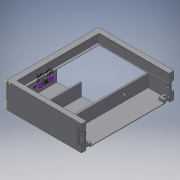
# Autodesk Inventor part: Bauteil1
Saved by Autodesk Inventor 2016 SP2 (Build 200236200, 236)
## iProperties
Created: 2018-06-21
Part Number: Bauteil1
Material: Generisch
Document SubType Name: Modeling
Designer: Nils
Density: 1 g/cm^3
Appearance: Vorgabe
Author: Nils
Autodesk Inventor part; units mm, degrees
ref_plane "YZ Plane" through (0, 0, 0) normal (1, 0, 0) x (0, 1, 0)
ref_plane "XZ Plane" through (0, 0, 0) normal (0, 1, 0) x (-1, 0, 0)
ref_plane "XY Plane" through (0, 0, 0) normal (0, 0, 1) x (1, 0, 0)
sketch "Skizze1" plane through (0, 0, 0) normal (0, 0, 1) x (1, 0, 0)
  line L0 (0, 0) -> (137.4, 0)
  line L1 (137.4, 0) -> (137.4, 9)
  line L2 (137.4, 9) -> (10, 9)
  line L3 (10, 9) -> (10, 159.5)
  line L4 (10, 159.5) -> (137.4, 159.5)
  line L5 (137.4, 159.5) -> (137.4, 168.5)
  line L6 (137.4, 168.5) -> (0, 168.5)
  line L7 (0, 168.5) -> (0, 0)
  dimension "d0" = 9
  dimension "d1" = 9
  dimension "d2" = 150.5
  dimension "d3" = 10
  dimension "d4" = 137.4
  constraints: 16 end point, 6 perpendicular, 2 point on line, 1 horizontal
  measures "d0" distance of L0.end L1.end
  measures "d1" distance of L4.end L5.end
  measures "d2" distance of L2.end L3.end
  measures "d3" distance between parallel lines of L7 L3
  measures "d4" distance of L0.start L0.end
extrude "Extrusion1" add sketch "Skizze1" along normal blind 1
sketch "Skizze2" plane through (0, 0, 0) normal (0, 0, -1) x (-1, 0, 0)
  line L0 (0, 0) -> (-137.4, 0) projected
  line L1 (0, 168.5) -> (0, 0) projected
  line L2 (-137.4, 168.5) -> (0, 168.5) projected
  line L3 (-137.4, 0) -> (-137.4, 4.5)
  line L4 (-137.4, 0) -> (-137.4, 9) projected
  line L5 (-6, 7.5) -> (-6, 161)
  line L6 (-10, 9) -> (-10, 159.5) projected
  line L7 (-6, 161) -> (-137.4, 161)
  line L8 (-137.4, 159.5) -> (-137.4, 168.5) projected
  line L9 (-137.4, 161) -> (-137.4, 168.5)
  line L10 (-10, 159.5) -> (-137.4, 159.5) projected
  line L11 (-6, 7.5) -> (-137.4, 7.5)
  line L12 (0, 0) -> (-137.4, 0) projected
  line L13 (-137.4, 7.5) -> (-137.4, 0)
  line L14 (-137.4, 9) -> (-10, 9) projected
  dimension "d7" = 1.5
  dimension "d8" = 1.5
  dimension "d9" = 4
  constraints: 12 end point, 2 parallel, 2 perpendicular, 2 point on line, 1 collinear, 1 midpoint
  measures "d7" distance between parallel lines of L10 L7
  measures "d8" distance between parallel lines of L14 L11
  measures "d9" distance between parallel lines of L6 L5
extrude "Extrusion2" add sketch "Skizze2" along normal blind 17 contours L0 L3 L4 L11 L5 L7 L8 L2 L1
sketch "Skizze3" plane through (0, 0, -17) normal (0, 0, -1) x (-1, 0, 0)
  line L0 (0, 0) -> (-137.4, 0) projected
  line L1 (-137.4, 0) -> (-137.4, 9) projected
  line L2 (-137.4, 9) -> (-10, 9) projected
  line L3 (-10, 9) -> (-10, 159.5) projected
  line L4 (-10, 159.5) -> (-137.4, 159.5) projected
  line L5 (-137.4, 159.5) -> (-137.4, 168.5) projected
  line L6 (-137.4, 168.5) -> (0, 168.5) projected
  line L7 (0, 168.5) -> (0, 0) projected
extrude "Extrusion3" add sketch "Skizze3" along normal blind 2
sketch "Skizze4" plane through (0, 0, -19) normal (0, 0, -1) x (-1, 0, 0)
  line L0 (-6, 161) -> (-137.4, 161) projected
  line L1 (-137.4, 161) -> (-6, 161) projected
  line L2 (-6, 7.5) -> (-6, 161) projected
  line L3 (-6, 161) -> (-6, 7.5) projected
  line L4 (-137.4, 7.5) -> (-6, 7.5) projected
  line L5 (-6, 7.5) -> (-137.4, 7.5) projected
  line L6 (0, 168.5) -> (-137.4, 168.5) projected
  line L7 (0, 0) -> (0, 168.5) projected
  line L8 (-137.4, 0) -> (0, 0) projected
  line L9 (0, 0) -> (-137.4, 0) projected
  line L10 (-137.4, 0) -> (-137.4, 7.5)
  line L11 (-137.4, 168.5) -> (-137.4, 159.5) projected
  line L12 (-137.4, 161) -> (-137.4, 168.5)
  line L13 (-137.4, 161) -> (-6, 161)
  line L14 (-6, 161) -> (-6, 7.5) projected
  line L15 (-6, 161) -> (-6, 7.5)
  line L16 (-137.4, 7.5) -> (-6, 7.5) projected
  line L17 (-6, 7.5) -> (-137.4, 7.5)
  constraints: 10 end point, 3 collinear, 2 perpendicular
extrude "Extrusion4" add sketch "Skizze4" along normal blind 23
sketch "Skizze5" plane through (0, 0, -42) normal (0, 0, -1) x (-1, 0, 0)
  line L0 (-137.4, 159.5) -> (-137.4, 168.5) projected
  line L1 (0, 0) -> (-137.4, 0) projected
  line L2 (-137.4, 168.5) -> (0, 168.5)
  line L3 (0, 168.5) -> (0, 0)
  line L4 (0, 0) -> (-137.4, 0)
  line L5 (-137.4, 0) -> (-137.4, 168.5)
  constraints: 8 end point, 2 parallel, 1 horizontal, 1 perpendicular
extrude "Extrusion5" add sketch "Skizze5" along normal blind 3
sketch "Skizze6" plane through (6, 7.5, -19) normal (0, 1, 0) x (1, 0, 0)
  line L0 (0, 0) -> (0, 23) projected
  line L1 (131.4, 0) -> (0, 0) projected
  line L2 (43.5, 0) -> (45.5, 0)
  line L3 (45.5, 0) -> (45.5, 23)
  line L4 (45.5, 23) -> (43.5, 23)
  line L5 (43.5, 23) -> (43.5, 0)
  line L6 (0, 23) -> (131.4, 23) projected
  line L7 (89, 23) -> (92, 23)
  line L8 (92, 23) -> (92, 0)
  line L9 (92, 0) -> (89, 0)
  line L10 (89, 0) -> (89, 23)
  point P0 (-6, -19)
  dimension "d24" = 43.5
  dimension "d25" = 43.5
  dimension "d26" = 2
  dimension "d27" = 3
  constraints: 16 end point, 4 parallel, 3 point on line, 2 horizontal, 2 perpendicular
  measures "d24" distance between parallel lines of L5 L0
  measures "d25" distance between parallel lines of L10 L3
  measures "d26" distance between parallel lines of L3 L5
  measures "d27" distance between parallel lines of L8 L10
chamfer "Fase2" distance 1.5 angle 45 2 edges at (73.7, 159.5, -19) (73.7, 9, -19)
chamfer "Fase3" distance 1.5 angle 45 1 edges at (10, 84.25, -19)
extrude "Extrusion7" add sketch "Skizze6" along normal blind 78.5 contours L5 L4 L3 L1 | L10 L6 L8 L1
sketch "Skizze7" plane through (0, 0, -42) normal (0, 0, 1) x (1, 0, 0)
  line L0 (137.4, 159.5) -> (10, 159.5) projected
  line L1 (98, 86) -> (96, 86)
  line L2 (137.4, 161) -> (6, 161) projected
  line L3 (98, 86) -> (95.5, 86)
  line L4 (95.5, 86) -> (95.5, 161)
  line L5 (95.5, 161) -> (98, 161)
  line L6 (98, 161) -> (98, 86)
  point P0 (0, 0)
  dimension "d46" = 2.5
  constraints: 10 end point, 2 horizontal, 2 parallel, 1 coincident, 1 perpendicular, 1 point on line
  measures "d46" distance of L4.end L5.end
extrude "Extrusion8" add sketch "Skizze7" along normal blind 23
sketch "Skizze8" plane through (0, 168.5, 1) normal (0, 1, 0) x (1, 0, 0)
  line L0 (95.5, 20) -> (95.5, 41) projected
  line L1 (0, 46) -> (95.5, 46)
  line L2 (95.5, 46) -> (95.5, 20)
  line L3 (95.5, 20) -> (0, 20)
  line L4 (0, 20) -> (0, 46)
  point P0 (0, 1)
  constraints: 8 end point, 2 parallel, 1 horizontal, 1 perpendicular
extrude "Extrusion9" cut sketch "Skizze8" against normal blind 82.5
sketch "Skizze9" plane through (95.5, 86, -45) normal (-1, 0, 0) x (0, 0, 1)
  line L0 (3, 0) -> (26, 0) projected
  line L1 (3, 0) -> (3, 1)
  line L2 (3, 75) -> (3, -78.5) projected
  line L3 (3, 1) -> (1, 1)
  line L4 (1, 1) -> (2, 0)
  line L5 (26, 0) -> (0, 0) projected
  line L6 (2, 0) -> (3, 0)
  point P0 (45, -86)
  dimension "d47" = 2
  dimension "d48" = 1
  dimension "d49" = 1
  constraints: 8 end point, 2 point on line, 1 collinear, 1 horizontal
  measures "d47" distance of L1.end L3.end
  measures "d48" distance of L0.start L1.end
  measures "d49" distance from line of L4.end L1
extrude "Extrusion10" add sketch "Skizze9" along normal blind 89.5
sketch "Skizze10" plane through (95.5, 86, -45) normal (-1, 0, 0) x (0, 0, 1)
  line L0 (26, 82.5) -> (26, 75) projected
  line L1 (26, 80.5) -> (25, 81.5)
  line L2 (25, 81.5) -> (25, 79.5)
  line L3 (25, 79.5) -> (26, 78.5)
  line L4 (26, 78.5) -> (26, 80.5)
  line L5 (0, 82.5) -> (26, 82.5) projected
  point P0 (45, -86)
  dimension "d52" = 2
  dimension "d53" = 1
  dimension "d54" = 2
  dimension "d55" = 1
  constraints: 8 end point, 2 parallel, 1 collinear, 1 point on line
  measures "d52" distance of L1.end L2.end
  measures "d53" distance from line of L0 L1.end
  measures "d54" distance of L1.start L0.start
  measures "d55" distance from line of L5 L1.end
extrude "Extrusion11" add sketch "Skizze10" along normal blind 89.5
sketch "Skizze11" plane through (0, 0, 1) normal (0, -1, 0) x (1, 0, 0)
  line L0 (0, 0) -> (137.4, 0) construction
  line L1 (129.4, 0) -> (129.4, -46) construction
  line L2 (95.5, -46) -> (137.4, -46) construction
  line L3 (137.4, -46) -> (137.4, 0) projected
  line L4 (137.4, -15) -> (129.4, -7)
  line L5 (129.4, -7) -> (129.4, -39)
  line L6 (129.4, -39) -> (137.4, -31)
  point P0 (0, -1)
  dimension "d58" = 15
  dimension "d59" = 15
  dimension "d60" = 8
  dimension "d61" = 8
  dimension "d62" = 8
  dimension "d63" = 16
  constraints: 8 end point, 6 point on line, 1 vertical
  measures "d58" distance of L2.end L6.end
  measures "d59" distance of L0.end L4.start
  measures "d60" distance between parallel lines of L1 L3
  measures "d61" horizontal distance of L5.end L6.end
  measures "d62" horizontal distance of L4.end L4.start
  measures "d63" distance of L6.end L4.start
extrude "Extrusion12" cut sketch "Skizze11" against normal blind 4.5
sketch "Skizze13" plane through (0, 4.5, 1) normal (0, -1, 0) x (1, 0, 0)
  line L0 (137.4, -15) -> (137.4, -31) projected
  line L1 (129.4, -7) -> (137.4, -15) projected
  line L2 (129.4, -39) -> (129.4, -7) projected
  line L3 (137.4, -31) -> (129.4, -39) projected
  line L4 (137.4, -20) -> (137.4, -43) construction
  line L5 (137.4, -23) -> (129.4, -23) construction
  circle A0 centre (133.4, -23) radius 1.75
  point P0 (0, -1)
  dimension "d66" = 3.5
  constraints: 2 end point, 2 midpoint, 1 centre point, 1 perpendicular, 1 point on line
  measures "d66" diameter of A0
extrude "Extrusion13" cut sketch "Skizze13" against normal blind 4.5 contours A0
sketch "Skizze14" plane through (137.4, 7.5, -19) normal (0, 1, 0) x (1, 0, 0)
  circle A0 centre (-4, 3) radius 1.75 construction
  line L0 (-5.6166, 5.8) -> (-2.3834, 5.8)
  line L1 (-2.3834, 5.8) -> (-0.7668, 3)
  line L2 (-0.7668, 3) -> (-2.3834, 0.2)
  line L3 (-2.3834, 0.2) -> (-5.6166, 0.2)
  line L4 (-5.6166, 0.2) -> (-7.2332, 3)
  line L5 (-7.2332, 3) -> (-5.6166, 5.8)
  point P0 (-137.4, -19)
  dimension "d69" = 5.6
  constraints: 12 end point, 1 coincident, 1 horizontal, 13 other
  measures "d69" distance between parallel lines of L2 L5
extrude "Extrusion14" cut sketch "Skizze14" against normal blind 2
chamfer "Fase4" distance 2 angle 5 1 edges at (130.9751, 7.5, -20.6) measured on face at (131.2446, 6.8333, -20.1333)
chamfer "Fase5" distance 2 angle 5 1 edges at (130.9751, 7.5, -23.4) measured on face at (131.2446, 6.1668, -23.8667)
chamfer "Fase6" distance 2 angle 5 1 edges at (133.4, 7.5, -24.8) measured on face at (133.9389, 6.1668, -24.8)
chamfer "Fase7" distance 2 angle 5 1 edges at (135.8249, 7.5, -23.4) measured on face at (136.0943, 6.1668, -22.9333)
chamfer "Fase9" distance 2 angle 5 1 edges at (133.4, 7.5, -19.2) measured on face at (133.9389, 6.1668, -19.2)
chamfer "Fase20" distance 2 angle 5 1 edges at (135.8249, 7.5, -20.6) measured on face at (136.0943, 6.167, -21.0667)
sketch "Skizze15" plane through (98, 7.5, -19) normal (1, 0, 0) x (0, 0, -1)
  line L0 (9, 108.5) -> (14, 108.5)
  line L1 (14, 108.5) -> (14, 113.5)
  line L2 (14, 113.5) -> (9, 113.5)
  line L3 (9, 113.5) -> (9, 108.5)
  line L4 (0, 153.5) -> (23, 153.5) projected
  line L5 (0, 153.5) -> (0, 78.5) projected
  point P0 (-19, -7.5)
  dimension "d90" = 5
  dimension "d91" = 5
  dimension "d92" = 40
  dimension "d93" = 9
  constraints: 8 end point, 2 parallel, 1 horizontal, 1 perpendicular
  measures "d90" distance of L2.end L1.end
  measures "d91" distance of L1.end L0.end
  measures "d92" distance from line of L4 L1.end
  measures "d93" distance between parallel lines of L5 L3
extrude "Extrusion15" cut sketch "Skizze15" against normal blind 40
sketch "Skizze16" plane through (0, 168.5, 1) normal (0, 1, 0) x (1, 0, 0)
  circle A0 centre (133.4, 23) radius 1.75 projected
  line L0 (137.4, 15) -> (137.4, 31) projected
  line L1 (129.4, 7) -> (137.4, 15) projected
  line L2 (129.4, 39) -> (129.4, 7) projected
  line L3 (137.4, 31) -> (129.4, 39) projected
  point P0 (0, 1)
extrude "Extrusion16" cut sketch "Skizze16" against normal blind 4.5
sketch "Skizze17" plane through (133.4, 168.5, -22) normal (0, 1, 0) x (1, 0, 0)
  circle A0 centre (0, 0) radius 1.75 projected
  point P0 (-133.4, -22)
extrude "Extrusion17" cut sketch "Skizze17" against normal blind 18
sketch "Skizze19" plane through (137.4, 161, -42) normal (0, -1, 0) x (1, 0, 0)
  circle A0 centre (-4, 20) radius 1.75 projected
  line L0 (-5.6166, 17.2) -> (-2.3834, 17.2) projected
  line L1 (-7.2332, 20) -> (-5.6166, 17.2) projected
  line L2 (-5.6166, 22.8) -> (-7.2332, 20) projected
  line L3 (-2.3834, 22.8) -> (-5.6166, 22.8) projected
  line L4 (-0.7668, 20) -> (-2.3834, 22.8) projected
  line L5 (-2.3834, 17.2) -> (-0.7668, 20) projected
  point P0 (-137.4, 42)
extrude "Extrusion18" cut sketch "Skizze19" against normal blind 2
chamfer "Fase14" distance 2 angle 5 1 edges at (130.9751, 161, -20.6) measured on face at (130.7057, 162.3333, -21.0667)
chamfer "Fase15" distance 2 angle 5 1 edges at (133.4, 161, -19.2) measured on face at (133.9389, 162.3332, -19.2)
chamfer "Fase16" distance 2 angle 5 1 edges at (135.8249, 161, -20.6) measured on face at (136.0943, 162.3332, -21.0667)
chamfer "Fase17" distance 2 angle 5 1 edges at (135.8249, 161, -23.4) measured on face at (135.5554, 162.3332, -23.8667)
chamfer "Fase18" distance 2 angle 5 1 edges at (133.4, 161, -24.8) measured on face at (132.8611, 162.3332, -24.8)
chamfer "Fase19" distance 2 angle 5 1 edges at (130.9751, 161, -23.4) measured on face at (130.7057, 161.6665, -22.9333)
sketch "Skizze21" plane through (0, 0, -45) normal (0, 0, -1) x (-1, 0, 0)
  line L0 (-98, 7.5) -> (-137.4, 7.5) projected
  line L1 (-137.4, 7.5) -> (-129.4, 7.5)
  line L2 (-129.4, 7.5) -> (-129.4, 161)
  line L3 (-6, 161) -> (-137.4, 161) projected
  line L4 (-137.4, 161) -> (-129.4, 161)
  line L5 (-137.4, 161) -> (-137.4, 7.5)
  point P0 (0, 0)
  dimension "d137" = 8
  constraints: 8 end point, 2 point on line, 1 collinear, 1 parallel, 1 perpendicular
  measures "d137" distance of L0.end L1.end
extrude "Extrusion20" cut sketch "Skizze21" against normal blind 2
sketch "Skizze22" plane through (0, 0, -42) normal (0, 0, 1) x (1, 0, 0)
  line L0 (137.4, 7.5) -> (127.4, 7.5)
  line L1 (127.4, 7.5) -> (127.4, 17.5)
  line L2 (127.4, 17.5) -> (137.4, 17.5)
  line L3 (137.4, 17.5) -> (137.4, 7.5)
  line L4 (137.4, 161) -> (127.4, 161)
  line L5 (127.4, 161) -> (127.4, 151)
  line L6 (127.4, 151) -> (137.4, 151)
  line L7 (137.4, 151) -> (137.4, 161)
  point P0 (0, 0)
  dimension "d140" = 10
  dimension "d141" = 10
  dimension "d142" = 10
  dimension "d143" = 10
  constraints: 16 end point, 4 parallel, 2 horizontal, 2 perpendicular
  measures "d140" distance of L1.end L2.end
  measures "d141" distance of L0.end L1.end
  measures "d142" distance of L6.end L5.end
  measures "d143" distance of L5.end L4.end
extrude "Extrusion21" add sketch "Skizze22" along normal blind 5
sketch "Skizze23" plane through (0, 0, -43) normal (0, 0, -1) x (-1, 0, 0)
  line L0 (-129.4, 161) -> (-129.4, 7.5) projected
  line L1 (-129.4, 7.5) -> (-137.4, 7.5)
  line L2 (-137.4, 7.5) -> (-137.4, 15.5)
  line L3 (-137.4, 15.5) -> (-129.4, 15.5)
  line L4 (-129.4, 15.5) -> (-129.4, 7.5)
  line L5 (-129.4, 161) -> (-137.4, 161)
  line L6 (-137.4, 161) -> (-137.4, 153)
  line L7 (-137.4, 153) -> (-129.4, 153)
  line L8 (-129.4, 153) -> (-129.4, 161)
  point P0 (0, 0)
  dimension "d146" = 8
  dimension "d147" = 8
  dimension "d148" = 8
  dimension "d149" = 8
  constraints: 16 end point, 4 parallel, 2 horizontal, 2 perpendicular
  measures "d146" distance of L2.end L3.end
  measures "d147" distance of L1.end L2.end
  measures "d148" distance of L7.end L6.end
  measures "d149" distance of L6.end L5.end
extrude "Extrusion22" cut sketch "Skizze23" against normal blind 2.5
sketch "Skizze24" plane through (0, 0, -40.5) normal (0, 0, -1) x (-1, 0, 0)
  line L0 (-137.4, 161) -> (-129.4, 161) projected
  line L1 (-137.4, 153) -> (-137.4, 161) projected
  line L2 (-129.4, 153) -> (-137.4, 153) projected
  line L3 (-129.4, 161) -> (-129.4, 153) projected
  line L4 (-129.4, 15.5) -> (-129.4, 7.5) projected
  line L5 (-137.4, 15.5) -> (-129.4, 15.5) projected
  line L6 (-137.4, 7.5) -> (-137.4, 15.5) projected
  line L7 (-129.4, 7.5) -> (-137.4, 7.5) projected
  line L8 (-137.4, 7.5) -> (-129.4, 15.5) construction
  line L9 (-137.4, 161) -> (-129.4, 153) construction
  circle A0 centre (-133.4, 157) radius 1.75
  circle A1 centre (-133.4, 11.5) radius 1.75
  point P0 (0, 0)
  dimension "d152" = 3.5
  dimension "d153" = 3.5
  constraints: 4 end point, 2 centre point, 2 midpoint, 1 perpendicular
  measures "d152" diameter of A0
  measures "d153" diameter of A1
extrude "Extrusion23" cut sketch "Skizze24" against normal blind 4.5 contours A0 | A1
sketch "Skizze25" plane through (0, 0, -37) normal (0, 0, 1) x (1, 0, 0)
  circle A0 centre (133.4, 157) radius 1.75 projected
  line L0 (136.3, 158.6743) -> (136.3, 155.3257)
  line L1 (136.3, 155.3257) -> (133.4, 153.6514)
  line L2 (133.4, 153.6514) -> (130.5, 155.3257)
  line L3 (130.5, 155.3257) -> (130.5, 158.6743)
  line L4 (130.5, 158.6743) -> (133.4, 160.3486)
  line L5 (133.4, 160.3486) -> (136.3, 158.6743)
  circle A1 centre (133.4, 11.5) radius 1.75 projected
  line L6 (130.5, 13.1743) -> (133.4, 14.8486)
  line L7 (133.4, 14.8486) -> (136.3, 13.1743)
  line L8 (136.3, 13.1743) -> (136.3, 9.8257)
  line L9 (136.3, 9.8257) -> (133.4, 8.1514)
  line L10 (133.4, 8.1514) -> (130.5, 9.8257)
  line L11 (130.5, 9.8257) -> (130.5, 13.1743)
  point P0 (0, 0)
  dimension "d156" = 5.8
  dimension "d157" = 5.8
  constraints: 24 end point, 2 coincident, 2 vertical, 26 other
  measures "d156" distance between parallel lines of L0 L3
  measures "d157" distance between parallel lines of L8 L11
extrude "Extrusion24" cut sketch "Skizze25" against normal blind 2.5
sketch "Skizze26" plane through (0, 0, 1) normal (-1, 0, 0) x (0, 0, 1)
  line L0 (-43, 86) -> (-20, 86) projected
  line L1 (-20, 86) -> (-46, 86) construction
  line L2 (-33, 86) -> (-33, 0) construction
  line L3 (-46, 0) -> (-31, 0) construction
  circle A0 centre (-33, 76) radius 1.75
  circle A1 centre (-33, 56) radius 1.75
  point P0 (-1, 0)
  dimension "d160" = 3.5
  dimension "d161" = 3.5
  dimension "d162" = 10
  dimension "d163" = 20
  constraints: 3 point on line, 2 centre point, 2 end point, 1 midpoint, 1 vertical
  measures "d160" diameter of A0
  measures "d161" diameter of A1
  measures "d162" distance from line of L0 A0.centre
  measures "d163" distance of A1.centre A0.centre
sketch "Skizze27" plane through (6, 7.5, -19) normal (1, 0, 0) x (0, 0, -1)
  circle A0 centre (13, 68.5) radius 1.75 projected
  circle A1 centre (13, 48.5) radius 1.75 projected
  line L0 (10.1, 66.8257) -> (10.1, 70.1743)
  line L1 (10.1, 70.1743) -> (13, 71.8486)
  line L2 (13, 71.8486) -> (15.9, 70.1743)
  line L3 (15.9, 70.1743) -> (15.9, 66.8257)
  line L4 (15.9, 66.8257) -> (13, 65.1514)
  line L5 (13, 65.1514) -> (10.1, 66.8257)
  line L6 (10.1, 46.8257) -> (10.1, 50.1743)
  line L7 (10.1, 50.1743) -> (13, 51.8486)
  line L8 (13, 51.8486) -> (15.9, 50.1743)
  line L9 (15.9, 50.1743) -> (15.9, 46.8257)
  line L10 (15.9, 46.8257) -> (13, 45.1514)
  line L11 (13, 45.1514) -> (10.1, 46.8257)
  point P0 (-19, -7.5)
  dimension "d166" = 5.8
  dimension "d167" = 5.8
  constraints: 24 end point, 2 coincident, 2 vertical, 26 other
  measures "d166" distance between parallel lines of L9 L6
  measures "d167" distance between parallel lines of L3 L0
sketch "Skizze28" plane through (0, 0, 1) normal (-1, 0, 0) x (0, 0, 1)
  line L0 (0, 0) -> (-46, 0) construction
  line L1 (-23, 0) -> (-23, 86) construction
  line L2 (-43, 86) -> (-20, 86) construction
  circle A0 centre (-23, 76) radius 5
  circle A1 centre (-23, 51) radius 5
  point P0 (-1, 0)
  dimension "d170" = 10
  dimension "d171" = 10
  dimension "d172" = 10
  dimension "d173" = 25
  constraints: 3 point on line, 2 centre point, 2 end point, 1 midpoint, 1 vertical
  measures "d170" diameter of A0
  measures "d171" diameter of A1
  measures "d172" distance from line of L2 A0.centre
  measures "d173" distance of A1.centre A0.centre
extrude "Extrusion27" cut sketch "Skizze28" against normal blind 5
thread "Gewinde3" size "M10x1.5" class "6H" standard "ANSI Metric M Profile" full length
thread "Gewinde4" size "M10x1.5" class "6H" standard "ANSI Metric M Profile" full length
sketch "Skizze34" plane through (5, 51, -22) normal (0, -1, 0) x (0, 0, 1)
  line L0 (5, 0) -> (5, 5)
  line L1 (5, 5) -> (4.0211, 5)
  line L2 (4.0211, 5) -> (4.0211, 0)
  line L3 (4.0211, 0) -> (5, 0)
  line L4 (0, -159.88) -> (0, 32.48) projected
  constraints: 8 end point
revolve "Umdrehung3" add sketch "Skizze34" angle 360 about axis through (5, 51, -22) along (-1, 0, 0) separate body
sketch "Skizze33" plane through (5, 51, -17) normal (0, 1, 0) x (-1, 0, 0)
  line L0 (-0.8887, -0.0802) -> (-0.7501, -0.0802) construction
  line L1 (0.1385, -0.899) -> (-0.0001, -1.1391) construction
  line L2 (-1.5001, -1.1391) -> (-1.6387, -0.899) construction
  line L3 (-0.6115, -0.0802) -> (-0.7501, 0.1599) construction
  line L4 (-0.7501, 0.1599) -> (-0.8887, -0.0802) construction
  line L5 (-1.5001, -1.1391) -> (-1.3615, -0.899) construction
  line L6 (-0.6115, -0.0802) -> (-0.1387, -0.899)
  line L7 (-1.6387, -0.899) -> (-1.3615, -0.899) construction
  arc A0 (-1.6387, -0.899) -> (-1.5001, -0.979) centre (-1.5001, -0.819) ccw construction
  line L8 (0.1385, -0.899) -> (-0.1387, -0.899) construction
  line L9 (-1.5001, -1.1391) -> (-1.5001, -0.899) construction
  line L10 (-0.0001, -1.1391) -> (-0.0001, -0.899) construction
  line L11 (-0.7501, 0.1599) -> (-0.7501, -0.0002) construction
  line L12 (-1.5001, -0.979) -> (-0.0001, -0.979)
  arc A1 (-1.5001, -0.979) -> (-1.3615, -0.899) centre (-1.5001, -0.819) ccw
  line L13 (-0.1387, -0.899) -> (-0.0001, -1.1391) construction
  line L14 (-1.3615, -0.899) -> (-0.8887, -0.0802)
  line L15 (-0.0001, -0.0002) -> (-0.0001, 0.0177)
  line L16 (-0.0001, 0.0177) -> (-0.0001, -0.0002)
  line L17 (-0.0001, -0.0002) -> (0.0334, -0.0002)
  arc A2 (-0.1387, -0.899) -> (-0.0001, -0.979) centre (-0.0001, -0.819) ccw
  arc A3 (-0.0001, -0.979) -> (0.1385, -0.899) centre (-0.0001, -0.819) ccw construction
  arc A4 (-0.7501, -0.0002) -> (-0.8887, -0.0802) centre (-0.7501, -0.1603) ccw
  arc A5 (-0.6115, -0.0802) -> (-0.7501, -0.0002) centre (-0.7501, -0.1603) ccw
  line L18 (-0.7501, -0.0002) -> (-0.7501, -0.0802) construction
  line L19 (-0.7501, -0.0802) -> (-0.6115, -0.0802) construction
  dimension "d220" = 60
  dimension "d221" = 0.2401
  dimension "d222" = 0.2401
  dimension "Skizze33_ThreadOffset" = 0
  dimension "Skizze33_MajorRadius" = 0.9789
  dimension "d225" = 1.5
  dimension "Skizze33_MinorRadius" = 0
  constraints: 40 end point, 12 point on circle, 10 parallel, 8 tangent, 6 centre point, 6 collinear, 2 midpoint, 2 point on line, 1 horizontal, 1 perpendicular, 3 other
  measures "d220" angle of L6 L14
  measures "d221" distance of L3.end L0.end
  measures "d222" distance of L1.end L10.end
  measures "Skizze33_ThreadOffset" distance between parallel lines of L15 L10
  measures "Skizze33_MajorRadius" distance from line of L12 L15.start
  measures "d225" distance from line of L1.end L9
  measures "Skizze33_MinorRadius" distance edge to line of A5 L17
coil "Spirale3" sketch "Skizze33" operation cut axis through (5, 51, -22) along (-1, 0, 0) pitch 1.5015 turns 5.328005 hand right bodies 2
sketch "Skizze36" plane through (5, 76, -22) normal (0, -1, 0) x (0, 0, 1)
  line L0 (5, 0) -> (5, 5)
  line L1 (5, 5) -> (4.0211, 5)
  line L2 (4.0211, 5) -> (4.0211, 0)
  line L3 (4.0211, 0) -> (5, 0)
  line L4 (0, -159.9745) -> (0, 33.0473) projected
  constraints: 8 end point
revolve "Umdrehung4" add sketch "Skizze36" angle 360 about axis through (5, 76, -22) along (-1, 0, 0) separate body
sketch "Skizze35" plane through (5, 76, -17) normal (0, 1, 0) x (-1, 0, 0)
  line L0 (-0.8887, -0.0802) -> (-0.7501, -0.0802) construction
  line L1 (0.1385, -0.899) -> (-0.0001, -1.1391) construction
  line L2 (-1.5001, -1.1391) -> (-1.6387, -0.899) construction
  line L3 (-0.6115, -0.0802) -> (-0.7501, 0.1599) construction
  line L4 (-0.7501, 0.1599) -> (-0.8887, -0.0802) construction
  line L5 (-1.5001, -1.1391) -> (-1.3615, -0.899) construction
  line L6 (-0.6115, -0.0802) -> (-0.1387, -0.899)
  line L7 (-1.6387, -0.899) -> (-1.3615, -0.899) construction
  arc A0 (-1.6387, -0.899) -> (-1.5001, -0.979) centre (-1.5001, -0.819) ccw construction
  line L8 (0.1385, -0.899) -> (-0.1387, -0.899) construction
  line L9 (-1.5001, -1.1391) -> (-1.5001, -0.899) construction
  line L10 (-0.0001, -1.1391) -> (-0.0001, -0.899) construction
  line L11 (-0.7501, 0.1599) -> (-0.7501, -0.0002) construction
  line L12 (-1.5001, -0.979) -> (-0.0001, -0.979)
  arc A1 (-1.5001, -0.979) -> (-1.3615, -0.899) centre (-1.5001, -0.819) ccw
  line L13 (-0.1387, -0.899) -> (-0.0001, -1.1391) construction
  line L14 (-1.3615, -0.899) -> (-0.8887, -0.0802)
  line L15 (-0.0001, -0.0002) -> (-0.0001, 0.0177)
  line L16 (-0.0001, 0.0177) -> (-0.0001, -0.0002)
  line L17 (-0.0001, -0.0002) -> (0.0334, -0.0002)
  arc A2 (-0.1387, -0.899) -> (-0.0001, -0.979) centre (-0.0001, -0.819) ccw
  arc A3 (-0.0001, -0.979) -> (0.1385, -0.899) centre (-0.0001, -0.819) ccw construction
  arc A4 (-0.7501, -0.0002) -> (-0.8887, -0.0802) centre (-0.7501, -0.1603) ccw
  arc A5 (-0.6115, -0.0802) -> (-0.7501, -0.0002) centre (-0.7501, -0.1603) ccw
  line L18 (-0.7501, -0.0002) -> (-0.7501, -0.0802) construction
  line L19 (-0.7501, -0.0802) -> (-0.6115, -0.0802) construction
  dimension "d238" = 60
  dimension "d239" = 0.2401
  dimension "d240" = 0.2401
  dimension "Skizze35_ThreadOffset" = 0
  dimension "Skizze35_MajorRadius" = 0.9789
  dimension "d243" = 1.5
  dimension "Skizze35_MinorRadius" = 0
  constraints: 40 end point, 12 point on circle, 10 parallel, 8 tangent, 6 centre point, 6 collinear, 2 midpoint, 2 point on line, 1 horizontal, 1 perpendicular, 3 other
  measures "d238" angle of L6 L14
  measures "d239" distance of L3.end L0.end
  measures "d240" distance of L1.end L10.end
  measures "Skizze35_ThreadOffset" distance between parallel lines of L15 L10
  measures "Skizze35_MajorRadius" distance from line of L12 L15.start
  measures "d243" distance from line of L1.end L9
  measures "Skizze35_MinorRadius" distance edge to line of A5 L17
coil "Spirale4" sketch "Skizze35" operation cut axis through (5, 76, -22) along (-1, 0, 0) pitch 1.5015 turns 5.328005 hand right bodies 3
equation "\"d1\" = d0"
equation "\"d8\" = d7"
equation "\"d25\" = d24"
equation "\"d59\" = d58"
equation "\"d61\" = d60"
equation "\"d62\" = d61"
equation "\"d94\" = d92"
equation "\"d220\" = d227"
equation "\"d221\" = 0.160083 * Skizze33_Pitch"
equation "\"d222\" = 0.160083 * Skizze33_Pitch"
equation "\"d225\" = Skizze33_Pitch"
equation "\"d238\" = d245"
equation "\"d239\" = 0.160083 * Skizze35_Pitch"
equation "\"d240\" = 0.160083 * Skizze35_Pitch"
equation "\"d243\" = Skizze35_Pitch"
equation "\"d187\" = 60deg"
equation "\"Skizze29_Pitch\" = 1.5"
equation "\"d205\" = 60deg"
equation "\"Skizze31_Pitch\" = 1.5"
equation "\"d227\" = 60deg"
equation "\"Skizze33_Pitch\" = 1.5"
equation "\"d245\" = 60deg"
equation "\"Skizze35_Pitch\" = 1.5"
